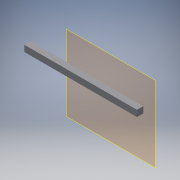
# Autodesk Inventor part: Intake Arm
Saved by Autodesk Inventor 2018 (Build 220112000, 112)
## iProperties
Created: 2018-01-18
Part Number: Intake Arm
Material: Generic
Document SubType Name: Modeling
Designer: Apple
Density: 1 g/cm^3
Appearance: Default
Author: Apple
Autodesk Inventor part; units mm, degrees
ref_plane "YZ Plane" through (0, 0, 0) normal (1, 0, 0) x (0, 1, 0)
ref_plane "XZ Plane" through (0, 0, 0) normal (0, 1, 0) x (-1, 0, 0)
ref_plane "XY Plane" through (0, 0, 0) normal (0, 0, 1) x (1, 0, 0)
ref_plane "Work Plane1" through (0, 0, 0) normal (0, 0, 1) x (1, 0, 0)
sketch "Sketch1" plane through (0, 0, 0) normal (0, 0, 1) x (1, 0, 0)
  line L0 (-165.1, -139.7) -> (165.1, -139.7) projected
  line L1 (-165.1, -139.7) -> (165.1, -139.7) construction
  line L2 (-325.7698, 38.3953) -> (131.4302, 38.3953)
  line L3 (131.4302, 38.3953) -> (131.4302, 12.9953)
  line L4 (131.4302, 12.9953) -> (-325.7698, 12.9953)
  line L5 (-325.7698, 12.9953) -> (-325.7698, 38.3953)
  point P0 (0, 0)
  dimension "d0" = 25.4
  dimension "d1" = 457.2
  constraints: 8 end point, 2 parallel, 1 horizontal, 1 perpendicular
  measures "d0" distance of L2.end L3.end
  measures "d1" distance of L2.start L2.end
extrude "Extrusion1" add sketch "Sketch1" along normal blind 25.4
sketch "Sketch2" plane through (-325.7698, 38.3953, 0) normal (0, 1, 0) x (1, 0, 0)
  circle A0 centre (14.9328, -13.0919) radius 4.7625
  point P0 (325.7698, 0)
  dimension "d4" = 9.525
  constraints: 1 centre point
  measures "d4" diameter of A0
extrude "Extrusion2" cut sketch "Sketch2" against normal through all
body "Solid1"
